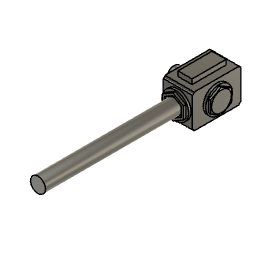
Piston Slider (Autodesk Fusion 360 design; units mm, degrees)
Autodesk Fusion 360 part; units mm, degrees
sketch "Sketch1" plane through (0, 0, 0) normal (0, 1, 0) x (1, 0, 0) in component "Component"
  line L0 (3, 0) -> (3, -2.5)
  line L1 (0, 3.45) -> (-1.45, 3.45)
  line L2 (1.45, -4.45) -> (-1.45, -4.45)
  line L3 (3.5, 2.5) -> (3.3905, 2.5)
  line L4 (2.1651, 1.25) -> (0, 2.5)
  line L5 (-1.45, 3.45) -> (-1.45, 4.45)
  line L6 (3.5, 0) -> (3.5, -2)
  line L7 (3, -2.5) -> (3.5, -2.5)
  line L8 (-3, 3.45) -> (0, 3.45)
  line L9 (1.45, 3.45) -> (1.45, 4.45)
  line L10 (-2.1651, -1.25) -> (0, -2.5)
  line L11 (4.5, -2) -> (3.5, -2)
  line L12 (0, -2.5) -> (2.1651, -1.25)
  line L13 (-1.7321, -1) -> (0, -2)
  line L14 (3.5, 2) -> (4.5, 2)
  line L15 (3, 2.5) -> (3.5, 2.5)
  line L16 (1.7321, 1) -> (0, 2)
  line L17 (0, 2.5) -> (-2.1651, 1.25)
  line L18 (-1.7321, 1) -> (-1.7321, -1)
  line L19 (3.5, 0) -> (3.5, 2)
  line L20 (-2.1651, 1.25) -> (-2.1651, -1.25)
  circle A0 centre (0, 0) radius 2.75
  line L21 (1.7321, -1) -> (1.7321, 1)
  line L22 (-3, -3.45) -> (-3, 3.45)
  line L23 (0, 3.45) -> (3, 3.45)
  line L24 (1.45, -3.45) -> (1.45, -4.45)
  line L25 (3.5, -2.5) -> (3.5, 2.5)
  line L26 (2.1651, -1.25) -> (2.1651, 1.25)
  line L27 (0, 3.45) -> (1.45, 3.45)
  line L28 (0, -3.45) -> (-3, -3.45)
  line L29 (3, -3.45) -> (0, -3.45)
  line L30 (4.5, 2) -> (4.5, -2)
  line L31 (3, 0) -> (3, 2.5)
  line L32 (-1.45, -3.45) -> (-1.45, -4.45)
  line L33 (-1.45, 4.45) -> (1.45, 4.45)
  line L34 (0, 2) -> (-1.7321, 1)
  circle A1 centre (0, 0) radius 1.55
  line L35 (3, 3.45) -> (3, -3.45)
  line L36 (0, -2) -> (1.7321, -1)
  dimension "d2" = 360
  dimension "d3" = 3.45
  dimension "d4" = 3.45
  dimension "d5" = 3
  dimension "d6" = 6.9
  dimension "d7" = 3
  dimension "d8" = 6.9
  dimension "d9" = 3
  dimension "d10" = 1.45
  dimension "d11" = 1.45
  dimension "d12" = 1
  dimension "d13" = 1
  dimension "d14" = 2.9
  dimension "d15" = 2.5
  dimension "d16" = 2.5
  dimension "d17" = 0.5
  dimension "d18" = 0.5
  dimension "d19" = 5
  dimension "d20" = 2
  dimension "d21" = 2
  dimension "d22" = 1
  dimension "d23" = 90
  dimension "d24" = 4
  dimension "d25" = 1
  dimension "d26" = 3.1
  dimension "d27" = 5.5
  dimension "d28" = 2
  dimension "d29" = 2.5
  constraint horizontal L23
  constraint vertical L35
  constraint horizontal L28
  constraint vertical L22
  constraint horizontal L8
  constraint parallel L23 L27
  constraint horizontal L1
  constraint vertical L9
  constraint vertical L5
  constraint perpendicular L9 L33
  constraint midpoint L0.start L35
  constraint perpendicular L1 L31
  constraint vertical L0
  constraint horizontal L15
  constraint horizontal L7
  constraint coincident L3.end L15
  constraint parallel L3 L15
  constraint vertical L25
  constraint vertical L19
  constraint midpoint L6.start L25
  constraint vertical L6
  constraint horizontal L14
  constraint horizontal L11
  constraint coincident A0.centre A1.centre
  measures "d3" distance of A0.centre L1.start
  measures "d4" distance of L28.start A0.centre
  measures "d5" distance of L23.end L1.start
  measures "d6" distance of L29.start L23.end
  measures "d7" distance of L28.start L22.start
  measures "d8" distance of L22.start L8.start
  measures "d9" distance of L1.start L8.start
  measures "d10" distance of L9.start L1.start
  measures "d11" distance of L1.end L1.start
  measures "d12" distance of L9.start L9.end
  measures "d13" distance of L5.end L1.end
  measures "d14" distance of L5.end L9.end
  measures "d15" distance of L0.start L15.start
  measures "d16" distance of L0.end L0.start
  measures "d17" distance of L3.start L15.start
  measures "d18" distance of L7.end L0.end
  measures "d19" distance of L7.end L3.start
  measures "d20" distance of L14.start L6.start
  measures "d21" distance of L6.end L6.start
  measures "d22" distance of L14.start L14.end
  measures "d23" angle of L14 L30
  measures "d24" distance of L11.start L14.end
  measures "d25" distance of L11.start L6.end
  measures "d26" diameter of A1
  measures "d27" diameter of A0
  measures "d28" distance of A0.centre L16.end
  measures "d29" distance of L4.end A0.centre
extrude "Extrude1" add sketch "Sketch1" along normal blind 10 contours L0 L1 L8 L22 L23 L27 L28 L29 L31 L35 | L2 L24 L28 L29 L32 | L1 L5 L8 L9 L23 L27 L33 | L4 L10 L12 L17 L20 L26 | L13 L16 L18 L21 L34 L36 | A0 | A1 in component "Component"
extrude "Extrude2" add sketch "Sketch1" against normal blind 0.5 contours A0 in component "Component"
extrude "Extrude3" add sketch "Sketch1" against normal blind 1 contours L4 L10 L12 L17 L20 L26 in component "Component"
extrude "Extrude4" add sketch "Sketch1" against normal blind 0.75 contours L13 L16 L18 L21 L34 L36 in component "Component"
extrude "Extrude5" add sketch "Sketch1" against normal blind 25 contours A1 in component "Component"
sketch "Sketch2" plane through (3, 0, 0) normal (1, 0, 0) x (0, 1, 0) in component "Component"
  line L0 (0, 3.45) -> (0, -3.45)
  line L1 (0, -3.45) -> (10, -3.45)
  line L2 (10, -3.45) -> (10, 3.45)
  line L3 (10, 3.45) -> (0, 3.45)
  circle A0 centre (5, 0) radius 2.75
  line L4 (5, -2.5) -> (7.1651, -1.25)
  line L5 (2.8349, -1.25) -> (5, -2.5)
  line L6 (2.8349, 1.25) -> (2.8349, -1.25)
  line L7 (5, 2.5) -> (2.8349, 1.25)
  line L8 (7.1651, 1.25) -> (5, 2.5)
  line L9 (7.1651, -1.25) -> (7.1651, 1.25)
  line L10 (5, -2) -> (6.7321, -1)
  line L11 (3.2679, -1) -> (5, -2)
  line L12 (3.2679, 1) -> (3.2679, -1)
  line L13 (5, 2) -> (3.2679, 1)
  line L14 (6.7321, 1) -> (5, 2)
  line L15 (6.7321, -1) -> (6.7321, 1)
  circle A1 centre (5, 0) radius 1.55
  dimension "d41" = 3.1
  dimension "d42" = 5.5
  dimension "d104" = 4
  dimension "d105" = 5
  measures "d41" diameter of A1
  measures "d42" diameter of A0
  measures "d104" distance of L13.start L10.start
  measures "d105" distance of L4.start L7.start
extrude "Extrude6" add sketch "Sketch2" along normal blind 1.5 contours L4 L5 L6 L7 L8 L9 in component "Component"
extrude "Extrude7" add sketch "Sketch2" along normal blind 0.5 contours A0 in component "Component"
extrude "Extrude8" cut 1 faces at (4.5, 6.299, -1.5833) along direction (-1, 0, 0) blind 0.5 in component "Component"
extrude "Extrude9" add sketch "Sketch2" along normal blind 1.5 contours A1 in component "Component"
extrude "Extrude10" add sketch "Sketch2" along normal blind 0.75 contours L10 L11 L12 L13 L14 L15 in component "Component"
extrude "Extrude11" cut sketch "Sketch1" along normal blind 10 contours L2 L24 L28 L29 L32 in component "Component"
extrude "Extrude12" add sketch "Sketch1" along normal blind 8.5 contours L2 L24 L28 L29 L32 in component "Component"
extrude "Extrude13" cut sketch "Sketch1" along normal blind 1.5 contours L2 L24 L28 L29 L32 in component "Component"
extrude "Extrude14" cut sketch "Sketch1" along normal blind 11 contours L1 L5 L8 L9 L23 L27 L33 in component "Component"
extrude "Extrude15" add sketch "Sketch1" along normal blind 8.5 contours L1 L5 L8 L9 L23 L27 L33 in component "Component"
extrude "Extrude16" cut sketch "Sketch1" along normal blind 1.5 contours L1 L5 L8 L9 L23 L27 L33 in component "Component"
extrude "Extrude17" cut 1 faces at (4.5, 5.5121, -0.5335) along direction (-1, 0, 0) blind 1.5 in component "Component"
extrude "Extrude18" cut 1 faces at (3, 5.5121, -0.5335) along direction (-1, 0, 0) blind 40.5 in component "Component"
extrude "Extrude19" cut 1 faces at (4, 6.299, -1.5833) along direction (-1, 0, 0) blind 0.5 in component "Component"
extrude "Extrude20" cut 1 faces at (3.75, 6.6714, 0) along direction (-1, 0, 0) blind 0.75 in component "Component"
extrude "Extrude21" add 1 faces at (3.5, 6.0357, 1.7939) along direction (-1, 0, 0) blind 7 in component "Component"
sketch "Sketch4" plane through (0, 0, 0) normal (1, 0, 0) x (0, 1, 0) in component "Component"
  line L0 (0, 0) -> (5, 0)
  line L1 (0, 0) -> (0, 3.45)
  line L2 (0, 0) -> (0, -3.45)
  line L3 (0, 3.45) -> (10, 3.45)
  line L4 (0, -3.45) -> (10, -3.45)
  line L5 (10, 3.45) -> (10, -3.45)
  circle A0 centre (0, 3.45) radius 0.375
  circle A1 centre (10, 3.45) radius 0.375
  circle A2 centre (0, -3.45) radius 0.375
  circle A3 centre (10, -3.45) radius 0.375
  dimension "d75" = 5
  dimension "d76" = 3.45
  dimension "d77" = 3.45
  dimension "d78" = 10
  dimension "d79" = 10
  dimension "d80" = 0.75
  dimension "d81" = 0.75
  dimension "d82" = 0.75
  dimension "d83" = 0.75
  constraint horizontal L0
  constraint coincident L0.start L1.start
  constraint vertical L1
  constraint vertical L2
  constraint horizontal L3
  constraint horizontal L4
  constraint coincident L1.end L3.start
  constraint coincident L3.end L5.start
  constraint coincident L2.end L4.start
  constraint coincident L4.end L5.end
  measures "d75" distance of L0.start L0.end
  measures "d76" distance of L0.start L1.end
  measures "d77" distance of L0.start L2.end
  measures "d78" distance of L1.end L3.end
  measures "d79" distance of L2.end L4.end
  measures "d80" diameter of A0
  measures "d81" diameter of A1
  measures "d82" diameter of A2
  measures "d83" diameter of A3
extrude "Extrude22" cut sketch "Sketch4" along normal mid plane 20 contours L1 L3 A0 | L2 L4 A2 | L3 L5 A1 | L4 L5 A3 picked at (0.2487, 3.4322) picked at (0.2336, -3.3629) picked at (9.7513, 3.4322) picked at (9.8237, -3.2737) in component "Component"
extrude "Extrude23" cut 1 faces at (0.8338, -25, 0.7144) along direction (0, 1, 0) blind 5 in component "Component"
extrude "Extrude24" add 1 faces at (0.8338, -20, 0.7144) along direction (0, -1, 0) blind 2.5 in component "Component"
extrude "Extrude25" add 1 faces at (0.8338, -22.5, 0.7144) along direction (0, -1, 0) blind 2.5 in component "Component"
extrude "Extrude26" cut 1 faces at (0.8338, -25, 0.7144) along direction (0, 1, 0) blind 2.5 in component "Component"
extrude "Extrude27" add 1 faces at (0.8338, -22.5, 0.7144) along direction (0, -1, 0) blind 1.25 in component "Component"
extrude "Extrude28" cut 1 faces at (3.5, 6.0357, 1.7939) along direction (-1, 0, 0) blind 1 in component "Component"
extrude "Extrude29" add 1 faces at (2.5, 6.0357, 1.7939) along direction (1, 0, 0) blind 0.5 in component "Component"
extrude "Extrude30" cut 1 faces at (-3.5, 6.0357, 1.7939) along direction (1, 0, 0) blind 1 in component "Component"
extrude "Extrude31" add 1 faces at (-2.5, 6.0357, 1.7939) along direction (-1, 0, 0) blind 0.5 in component "Component"
extrude "Extrude32" add sketch "Sketch2" along normal blind 1 contours L4 L5 L6 L7 L8 L9 | L10 L11 L12 L13 L14 L15 | A1 in component "Component"
extrude "Extrude33" add sketch "Sketch2" along normal blind 0.5 contours A0 in component "Component"
sketch "Sketch1 (2)" plane through (0, 0, 0) normal (0, 0, 1) x (1, 0, 0)
  line L0 (4, 7.05) -> (3.8006, 8.0299)
  line L1 (4, 7.05) -> (3, 7.05) construction
  line L2 (3.8006, 8.0299) -> (4, 8.0299)
  line L3 (4, 8.0299) -> (4, 7.05)
  dimension "d110" = 78.5
  dimension "d111" = 1
  constraint horizontal L1
  constraint horizontal L2
  constraint perpendicular L2 L3
  measures "d110" angle of L0 L1
  measures "d111" distance of L0.start L0.end
revolve "Revolve1" cut sketch "Sketch1 (2)" angle 360 about axis through (3, 5, 0) along (-1, 0, 0) in component "Component"
extrude "Extrude34" add sketch "Sketch2" against normal blind 6.1 contours A1 in component "Component"
extrude "Extrude35" add 1 faces at (-3.1, 5.5121, -0.5335) along direction (-1, 0, 0) blind 8.75 in component "Component"
extrude "Extrude36" cut 1 faces at (-11.85, 5.5121, -0.5335) along direction (1, 0, 0) blind 0.1 in component "Component"
extrude "Extrude37" cut 1 faces at (-11.75, 5.5121, -0.5335) along direction (1, 0, 0) blind 14.75 in component "Component"
extrude "Extrude38" add 1 faces at (3, 5.5121, -0.5335) along direction (-1, 0, 0) blind 8.75 in component "Component"
extrude "Extrude39" cut 1 faces at (-5.75, 5.5121, -0.5335) along direction (1, 0, 0) blind 2.75 in component "Component"
sketch "Sketch2 (2)" plane through (-3, 0, 0) normal (-1, 0, 0) x (0, -1, 0)
  arc A0 (-10, 3.075) -> (-9.625, 3.45) centre (-10, 3.45) ccw
  line L0 (-10, 3.075) -> (-10, -3.075)
  arc A1 (-9.625, -3.45) -> (-10, -3.075) centre (-10, -3.45) ccw
  line L1 (-9.625, -3.45) -> (-0.375, -3.45)
  arc A2 (0, -3.075) -> (-0.375, -3.45) centre (0, -3.45) ccw
  line L2 (0, -3.075) -> (0, 3.075)
  arc A3 (-0.375, 3.45) -> (0, 3.075) centre (0, 3.45) ccw
  line L3 (-0.375, 3.45) -> (-9.625, 3.45)
  line L4 (0, 0) -> (-5, 0)
  circle A4 centre (-5, 0) radius 1.5
  dimension "d125" = 5
  dimension "d126" = 3
  constraint coincident L4.start origin
  constraint perpendicular L2 L4
  constraint coincident L4.end A4.centre
  measures "d125" distance of L4.start L4.end
  measures "d126" diameter of A4
extrude "Extrude40" cut sketch "Sketch2 (2)" against normal blind 6 contours A4 in component "Component"
extrude "Extrude41" add 1 faces at (3, 5.7249, 0.1093) along direction (-1, 0, 0) blind 8.75 in component "Component"
extrude "Extrude42" add 1 faces at (0.8338, -23.75, 0.7144) along direction (0, -1, 0) blind 5 in component "Component"
component "Component" placed x (1, 0, 0) y (0, 1, 0) z (0, 0, 1) at (0, 0, 0)
equation "d110 = 90 deg - 11.5 deg"
equation "d119 = -8.75 mm - 6 mm"
